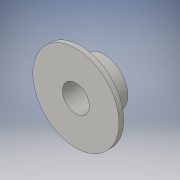
# Autodesk Inventor part: bearing
Saved by Autodesk Inventor 2016 (Build 200138000, 138)
## iProperties
Created: 2019-02-22
Part Number: bearing
Material: Generic
Document SubType Name: Modeling
Designer: reesem783
Density: 1 g/cm^3
Appearance: Default
Author: reesem783
Autodesk Inventor part; units mm, degrees
ref_plane "YZ Plane" through (0, 0, 0) normal (1, 0, 0) x (0, 1, 0)
ref_plane "XZ Plane" through (0, 0, 0) normal (0, 1, 0) x (-1, 0, 0)
ref_plane "XY Plane" through (0, 0, 0) normal (0, 0, 1) x (1, 0, 0)
sketch "Sketch1" plane through (0, 0, 0) normal (1, 0, 0) x (0, 1, 0)
  line L0 (0.019, 0.9702) -> (3.175, 0.9702)
  line L1 (3.175, 0.9702) -> (3.175, -2.1413)
  line L2 (0.019, 9.2838) -> (0.019, -29.9451)
  line L3 (3.175, -2.1413) -> (0.019, -2.1413)
  point P0 (0, 0)
  dimension "d3" = 3.1559
  dimension "d4" = 3.1115
  constraints: 8 end point, 2 perpendicular, 2 point on line, 1 horizontal
  measures "d3" distance of L0.start L0.end
  measures "d4" distance of L0.end L1.end
revolve "Revolution1" add sketch "Sketch1" angle 360 about axis through (0, 0.019, 9.2838) along (0, 0, -1)
sketch "Sketch3" plane through (0, 0.019, 0.9702) normal (0, 0, 1) x (1, 0, 0)
  circle A0 centre (0, 0) radius 5.715
  point P0 (0, -0.019)
  constraints: 1 centre point
extrude "Extrusion2" add sketch "Sketch3" along normal blind 0.635
sketch "Sketch4" plane through (0, 0.019, 1.6052) normal (0, 0, 1) x (1, 0, 0)
  point P0 (0, -0.019)
  point P1 (0, -0.019)
  constraints: 1 coincident
hole "Hole2" at (0, 0, 1.6052) direction (0, 0, -1) diameter 3.556 end through all
body "Solid1"
